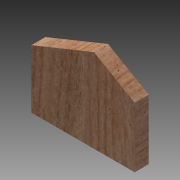
# Autodesk Inventor part: side battery
Saved by Autodesk Inventor 2014 (Build 180170000, 170)
## iProperties
Created: 2016-02-01
Part Number: side battery
Material: Generic
Document SubType Name: Modeling
Designer: sametj
Density: 1 g/cm^3
Appearance: Default
Author: sametj
Autodesk Inventor part; units mm, degrees
ref_plane "YZ Plane" through (0, 0, 0) normal (1, 0, 0) x (0, 1, 0)
ref_plane "XZ Plane" through (0, 0, 0) normal (0, 1, 0) x (-1, 0, 0)
ref_plane "XY Plane" through (0, 0, 0) normal (0, 0, 1) x (1, 0, 0)
sketch "Sketch1" plane through (0, 0, 0) normal (0, 0, 1) x (1, 0, 0)
  line L0 (-5.7054, 0) -> (133.9946, 0)
  line L1 (133.9946, 0) -> (133.9946, 81.28)
  line L2 (133.9946, 81.28) -> (79.002, 113.03)
  line L3 (-5.7054, 0) -> (-5.7054, 78.74)
  line L4 (-5.7054, 78.74) -> (79.002, 113.03)
  point P0 (0, 0)
  dimension "d0" = 139.7
  dimension "d1" = 81.28
  dimension "d2" = 63.5
  dimension "d3" = 120
  dimension "d4" = 78.74
  constraints: 10 end point, 1 horizontal, 1 parallel, 1 perpendicular
  measures "d0" distance of L0.start L0.end
  measures "d1" distance of L0.end L1.end
  measures "d2" distance of L1.end L2.end
  measures "d3" angle of L2 L1
  measures "d4" distance of L0.start L3.end
extrude "Extrusion1" add sketch "Sketch1" along normal blind 19.05
body "Solid1"
